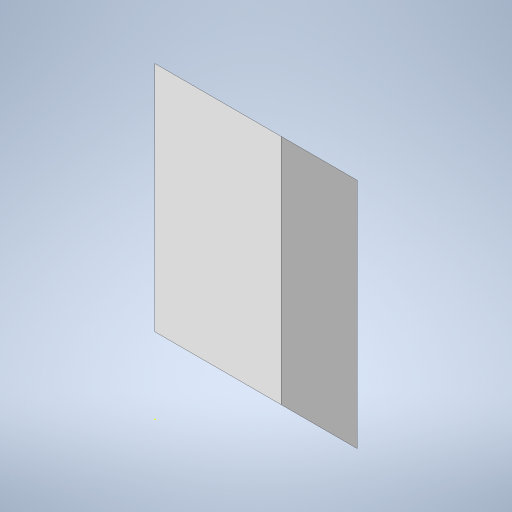
# Autodesk Inventor part: Mordaza
Saved by Autodesk Inventor 2023 (Build 270158000, 158)
## iProperties
Created: 2023-11-09
Part Number: Mordaza
Material: Genérico
Document SubType Name: Modeling
Designer: JULIAN
Density: 1 g/cm^3
Appearance: Valor por defecto
Author: JULIAN
Autodesk Inventor part; units mm, degrees
ref_plane "YZ Plane" through (0, 0, 0) normal (1, 0, 0) x (0, 1, 0)
ref_plane "XZ Plane" through (0, 0, 0) normal (0, 1, 0) x (-1, 0, 0)
ref_plane "XY Plane" through (0, 0, 0) normal (0, 0, 1) x (1, 0, 0)
sketch "Boceto1" plane through (0, 0, 0) normal (1, 0, 0) x (0, 1, 0)
  line L0 (9.1924, 0) -> (0, 0)
  line L1 (12.1924, 3) -> (9.1924, 0)
  line L2 (3, 3) -> (12.1924, 3)
  line L3 (0, 0) -> (3, 3)
  constraints: 8 end point
extrude "Extrusión1" add sketch "Boceto1" along normal blind 5
sketch "Boceto2" plane through (0, 3, 3) normal (0, 0, 1) x (1, 0, 0)
  point P0 (0, -3)
